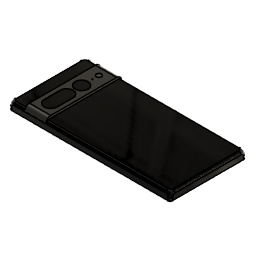
Pixel 7 Pro (Autodesk Fusion 360 design; units mm, degrees)
Autodesk Fusion 360 part; units mm, degrees
sketch "Sketch1" plane through (0, 0, 0) normal (0, 0, 1) x (1, 0, 0)
  line L0 (0, 0) -> (162.9, 0)
  line L1 (162.9, 0) -> (162.9, 76.6)
  line L2 (162.9, 76.6) -> (0, 76.6)
  line L3 (0, 76.6) -> (0, 0)
  dimension "d1" = 162.9
  dimension "d2" = 76.6
  constraint horizontal L0
  constraint vertical L1
  constraint horizontal L2
  constraint vertical L3
  constraint coincident L0.start L3.end
  measures "d1" distance of L0.start L0.end
  measures "d2" distance of L0.start L2.end
extrude "Extrude1" add sketch "Sketch1" along normal blind 8.9 makes body 1
move_body "Move1" bodies 1 to x (1, 0, 0) y (0, 1, 0) z (0, 0, 1) at (-1, 0, 0)
sketch "Sketch2" plane through (0, 0, 8.9) normal (0, 0, 1) x (-1, 0, 0)
  line L0 (1, -76.6) -> (1, 0)
  line L1 (1, 0) -> (-161.9, 0)
  line L2 (-161.9, 0) -> (-161.9, -76.6)
  line L3 (-161.9, -76.6) -> (1, -76.6)
  line L4 (-14.508, 0) -> (-36.0413, 0)
  line L5 (-36.0413, 0) -> (-36.0413, -76.6)
  line L6 (-36.0413, -76.6) -> (-14.508, -76.6)
  line L7 (-14.508, -76.6) -> (-14.508, 0)
  line L8 (-25.2746, 0) -> (-25.2746, -76.6) construction
  circle A0 centre (-25.2746, -64.5081) radius 2.5
  circle A1 centre (-25.2746, -57.8882) radius 0.5
  circle A2 centre (-25.2746, -47.0052) radius 2
  circle A3 centre (-25.2746, -47.0052) radius 6.5
  circle A4 centre (-25.2746, -31.8825) radius 1.5
  circle A5 centre (-25.2746, -31.8825) radius 3
  circle A6 centre (-25.2746, -15.7564) radius 2
  circle A7 centre (-25.2746, -15.7564) radius 3
  line L9 (-25.2746, -31.8825) -> (-31.7746, -31.8825) construction
  line L10 (-31.7746, -31.8825) -> (-31.7746, -15.7564)
  line L11 (-18.7746, -31.8825) -> (-18.7746, -15.7564)
  arc A8 (-31.7746, -31.8825) -> (-18.7746, -31.8825) centre (-25.2746, -31.8825) ccw
  arc A9 (-18.7746, -15.7564) -> (-31.7746, -15.7564) centre (-25.2746, -15.7564) ccw
  dimension "d5" = 5
  dimension "d6" = 1
  dimension "d7" = 4
  dimension "d8" = 13
  dimension "d9" = 3
  dimension "d10" = 6
  dimension "d11" = 13
  dimension "d12" = 4
  dimension "d13" = 6
  dimension "d14" = 13
  constraint horizontal L4
  constraint vertical L5
  constraint horizontal L6
  constraint vertical L7
  constraint coincident L3 L5.end
  constraint coincident L1 L4.start
  constraint midpoint L4 L8.start
  constraint midpoint L6 L8.end
  constraint coincident L8 A0.centre
  constraint coincident L8 A1.centre
  constraint coincident L8 A2.centre
  constraint concentric A2 A3
  constraint coincident L8 A4.centre
  constraint concentric A4 A5
  constraint concentric A4 A8
  constraint coincident L8 A6.centre
  constraint concentric A6 A7
  constraint concentric A7 A9
  constraint coincident A4.centre A5.centre
  constraint perpendicular L8 L9
  constraint tangent L10 A9
  constraint perpendicular L9 L10
  constraint symmetric L8 L9.end L11.start
  constraint symmetric L8 L10.end L11.end
  measures "d5" diameter of A0
  measures "d6" diameter of A1
  measures "d7" diameter of A2
  measures "d8" diameter of A3
  measures "d9" diameter of A4
  measures "d10" diameter of A5
  measures "d11" diameter of A8
  measures "d12" diameter of A6
  measures "d13" diameter of A7
  measures "d14" diameter of A9
extrude "Extrude2" cut sketch "Sketch2" against normal blind 3 contours L0 L1 L3 L7 | L1 L2 L3 L5 bodies 1
extrude "Extrude3" add 1 faces at (53.3, 51.0667, 0) along direction (0, 0, -1) blind 3 on bodies 1 bodies 1
extrude "Extrude4" add 2 faces at (4.1693, 51.0667, 5.9) (77.9942, 51.0667, 5.9) along direction (0, 0, 1) blind 0.5 on bodies 1 bodies 1
extrude "Extrude5" cut 1 faces at (53.3, 51.0667, -3) along direction (0, 0, 1) blind 0.5 on bodies 1 bodies 1
extrude "Extrude6" add sketch "Sketch2" against normal blind 0.25 separate body contours A0 | A1 | A2 | A3 | A4 | A5 | A6 | A7 | L10 L11 A8 A9 makes body 2 at (23.108, 26.5071, 8.9) makes body 3 at (26.0419, 63.838, 8.9) makes body 4 at (23.3225, 47.9453, 8.9) makes body 5 at (25.2376, 58.1003, 8.9)
combine "Combine1" operation cut target body 1 tool bodies 2 3 5 4 keep tools
fillet "Fillet1" radius 2.5 10 edges at (98.9707, 0, 6.4) (6.754, 0, 6.4) (-1, 0, 1.95) (-1, 38.3, 6.4) (6.754, 76.6, 6.4) (98.9707, 76.6, 6.4) (161.9, 38.3, 6.4) (161.9, 0, 1.95) (-1, 76.6, 1.95) (161.9, 76.6, 1.95) on bodies 1
fillet "Fillet2" radius 5 2 edges at (25.2746, 76.6, 8.9) (25.2746, 0, 8.9) on bodies 1
fillet "Fillet3" radius 1 8 edges at (-1, 38.3, -2.5) (-0.2678, 0.7322, -2.5) (80.45, 0, -2.5) (161.1678, 0.7322, -2.5) (161.9, 38.3, -2.5) (161.1678, 75.8678, -2.5) (80.45, 76.6, -2.5) (-0.2678, 75.8678, -2.5) on bodies 1
sketch "Sketch3" plane through (0, 0, -2.5) normal (0, 0, -1) x (1, 0, 0)
  line L0 (0, -2.5) -> (0, -74.1)
  arc A0 (0, -74.1) -> (1.5, -75.6) centre (1.5, -74.1) ccw
  line L1 (1.5, -75.6) -> (159.4, -75.6)
  arc A1 (159.4, -75.6) -> (160.9, -74.1) centre (159.4, -74.1) ccw
  line L2 (160.9, -74.1) -> (160.9, -2.5)
  arc A2 (160.9, -2.5) -> (159.4, -1) centre (159.4, -2.5) ccw
  line L3 (159.4, -1) -> (1.5, -1)
  arc A3 (1.5, -1) -> (0, -2.5) centre (1.5, -2.5) ccw
  line L4 (-14.8095, -96.0954) -> (176.6898, -96.0954)
  line L5 (176.6898, -96.0954) -> (176.6898, 31.5708)
  line L6 (176.6898, 31.5708) -> (-14.8095, 31.5708)
  line L7 (-14.8095, 31.5708) -> (-14.8095, -96.0954)
  constraint horizontal L4
  constraint vertical L5
  constraint horizontal L6
  constraint vertical L7
copy_body "CopyPasteBodies1" bodies 1 makes body 6
extrude "Extrude7" cut sketch "Sketch3" 1 faces at (54.1333, 25.8667, -2.5) against normal blind 1 keep common part on bodies 1 bodies 1
combine "Combine2" operation cut target body 6 tool bodies 1 keep tools
extrude "Extrude8" add 1 faces at (36.0413, 27.2, 7.2333) along direction (-1, 0, 0) blind 21.533 separate body on bodies 6 makes body 7
combine "Combine3" operation cut target body 6 tool bodies 7 keep tools
combine "Combine4" operation cut target body 7 tool bodies 2 4 3 5 keep tools
ref_plane "WorkPlane1" through (0, 76.6, 0) normal (0, 1, 0) x (0, 0, 1)
sketch "Sketch4" plane through (0, 0, 0) normal (0, 1, 0) x (1, 0, 0)
  line L0 (52, -36, 76.6) -> (52, -2, 76.6) construction
  line L1 (63, -36, 76.6) -> (63, -2, 76.6) construction
  line L2 (73, -36, 76.6) -> (73, -2, 76.6) construction
  line L3 (93.669, -36, 76.6) -> (93.669, -2, 76.6) construction
  line L4 (52, -2, 76.6) -> (93.669, -2, 76.6)
  line L5 (52, -2, 76.6) -> (63, -2, 76.6)
  line L6 (61.7496, -0.75, 76.6) -> (53.2504, -0.75, 76.6)
  line L7 (52.0005, -1.9999, 76.6) -> (52.0005, -2.0001, 76.6)
  line L8 (53.2504, -3.25, 76.6) -> (61.7496, -3.25, 76.6)
  line L9 (62.9995, -2.0001, 76.6) -> (62.9995, -1.9999, 76.6)
  line L10 (62.9995, -0.75, 76.6) -> (52.0005, -3.25, 76.6) construction
  line L11 (52.0005, -0.75, 76.6) -> (62.9995, -3.25, 76.6) construction
  arc A0 through (52.0005, -2.0001, 76.6) (52.3666, -2.8839, 76.6) (53.2504, -3.25, 76.6)
  arc A1 through (61.7496, -3.25, 76.6) (62.6334, -2.8839, 76.6) (62.9995, -2.0001, 76.6)
  arc A2 through (62.9995, -1.9999, 76.6) (62.6334, -1.1161, 76.6) (61.7496, -0.75, 76.6)
  arc A3 through (53.2504, -0.75, 76.6) (52.3666, -1.1161, 76.6) (52.0005, -1.9999, 76.6)
  line L12 (73, -2, 76.6) -> (93.669, -2, 76.6)
  line L13 (92.4191, -3.25, 76.6) -> (74.2499, -3.25, 76.6)
  line L14 (73, -2.0001, 76.6) -> (73, -1.9999, 76.6)
  line L15 (74.2499, -0.75, 76.6) -> (92.4191, -0.75, 76.6)
  line L16 (93.669, -1.9999, 76.6) -> (93.669, -2.0001, 76.6)
  line L17 (93.669, -3.25, 76.6) -> (73, -0.75, 76.6) construction
  line L18 (73, -3.25, 76.6) -> (93.669, -0.75, 76.6) construction
  arc A4 through (92.4191, -3.25, 76.6) (93.3029, -2.8839, 76.6) (93.669, -2.0001, 76.6)
  arc A5 through (93.669, -1.9999, 76.6) (93.3029, -1.1161, 76.6) (92.4191, -0.75, 76.6)
  arc A6 through (74.2499, -0.75, 76.6) (73.3661, -1.1161, 76.6) (73, -1.9999, 76.6)
  arc A7 through (73, -2.0001, 76.6) (73.3661, -2.8839, 76.6) (74.2499, -3.25, 76.6)
  point P0 (57.5, -2)
  point P1 (83.3345, -2)
  dimension "d36" = 2.5
  dimension "d37" = 1.2499
  dimension "d38" = 2.5
  dimension "d39" = 1.2499
extrude "Extrude9" add sketch "Sketch4" along normal blind 1 contours L4 L5 L6 A2 A3 | L4 L5 L8 A0 A1 | L4 L12 L15 A5 A6 | L4 L12 L13 A4 A7 in plane through (0, 76.6, 0) normal (0, 1, 0) bodies 6
